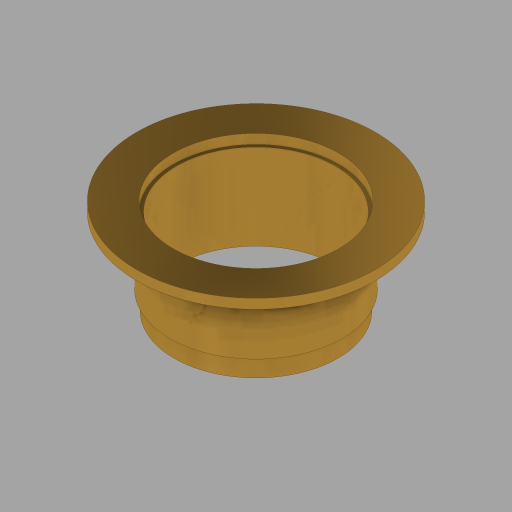
# Autodesk Inventor part: neckForStorage
Saved by Autodesk Inventor 2024 (Build 280153020, 153B)
## iProperties
Created: 2023-11-04
Part Number: neckForStorage
Material: Brass
Document SubType Name: Modeling
Designer: schanen
Density: 8.49 g/cm^3
Appearance: Brass - Polished
Mass: 138.614 g
Surface Area: 114.103 cm^2
Volume: 16.3653 cm^3
neck_ir: 25.000 mm
Author: schanen
Autodesk Inventor part; units mm, degrees
ref_plane "YZ Plane" through (0, 0, 0) normal (1, 0, 0) x (0, 1, 0)
ref_plane "XZ Plane" through (0, 0, 0) normal (0, 1, 0) x (-1, 0, 0)
ref_plane "XY Plane" through (0, 0, 0) normal (0, 0, 1) x (1, 0, 0)
sketch "Sketch1" plane through (0, 0, 0) normal (0, 0, 1) x (1, 0, 0)
  line L0 (-25, 27) -> (-25, 0)
  line L1 (-25, 0) -> (-25.75, 0)
  line L2 (-25.75, 0) -> (-25.75, 6)
  line L3 (-25.75, 6) -> (-27, 6)
  line L4 (-27, 6) -> (-27, 24.1865)
  line L5 (-37.5, 30) -> (-26, 30)
  line L6 (-26, 30) -> (-26, 27)
  line L7 (-26, 27) -> (-25, 27)
  line L8 (0, -6) -> (0, 36) projected
  line L9 (-37.5, 30) -> (-37.5, 27)
  line L10 (-37.5, 27) -> (-27, 24.1865)
  point P0 (0, 0)
  dimension "d0" = 25.75
  dimension "neck_ir" = 25
  dimension "d5" = 6
  dimension "d15" = 27
  dimension "d16" = 3
  dimension "d17" = 37.5
  dimension "d18" = 26
  dimension "d19" = 15
  dimension "d20" = 3
  dimension "d21" = 30
  constraints: 20 end point, 6 perpendicular, 2 vertical, 1 horizontal alignment
  measures "d0" distance from line of point (0, 0) L2
  measures "neck_ir" distance from line of point (0, 0) L0
  measures "d5" distance of L1.end L2.end
  measures "d15" distance from line of point (0, 0) L4
  measures "d16" distance of L5.start L9.end
  measures "d17" distance between parallel lines of L8 L9
  measures "d18" distance between parallel lines of L8 L6
  measures "d19" angle of L10 L5
  measures "d20" distance of L5.end L6.end
  measures "d21" distance from line of point (0, 0) L5
revolve "Revolution1" add sketch "Sketch1" angle 360 about axis through (0, -10, 0) along (0, 1, 0)
equation "\"oring_diameter\" = 4"
body "Solid1"
